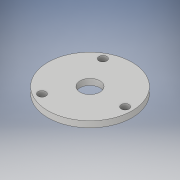
# Autodesk Inventor part: disk-sheet-b
Saved by Autodesk Inventor 2019.4 (Build 234330000, 330)
## iProperties
Created: 2020-04-05
Part Number: disk-sheet-b
Material: Generic
Document SubType Name: Sheet Metal
Designer: Phil
Density: 1 g/cm^3
Sheet Metal Rule: Default
Appearance: Default
Sheet Metal Width: 1.650 in
Sheet Metal Length: 1.650 in
Sheet Metal Area: 2.723 in^2
Flat Pattern Width: 4.191 cm
Flat Pattern Length: 4.191 cm
Flat Pattern Area: 17.5645 cm^2
Author: Phil
Autodesk Inventor part; units mm, degrees
ref_plane "YZ Plane" through (0, 0, 0) normal (1, 0, 0) x (0, 1, 0)
ref_plane "XZ Plane" through (0, 0, 0) normal (0, 1, 0) x (-1, 0, 0)
ref_plane "XY Plane" through (0, 0, 0) normal (0, 0, 1) x (1, 0, 0)
sketch "Sketch1" plane through (0, 0, 0) normal (0, 1, 0) x (-1, 0, 0)
  circle A0 centre (0, 0) radius 20.955
  circle A1 centre (0, 0) radius 4.9606
  circle A2 centre (-17.5514, 0) radius 1.9812
  circle A3 centre (8.7757, -15.2) radius 1.9812
  circle A4 centre (8.7757, 15.2) radius 1.9812
  dimension "d0" = 41.91
  dimension "d1" = 9.9212
  dimension "d2" = 3.9624
  dimension "d5" = 360
  measures "d0" diameter of A0
  measures "d1" diameter of A1
  measures "d2" diameter of A2
extrude "Plate1" add sketch "Sketch1" along normal blind 3.048
equation "\"d7\" = Thickness"
equation "\"BendRadius\" = Thickness"
equation "\"BendReliefWidth\" = Thickness"
equation "\"BendReliefDepth\" = 0.5 * Thickness"
equation "\"CornerReliefSize\" = 4 * Thickness"
equation "\"MinimumRemnant\" = 2 * Thickness"
equation "\"TransitionRadius\" = BendRadius"
equation "\"JacobiRadiusSize\" = BendRadius"
equation "\"GapSize\" = Thickness"
equation "\"Thickness\" = 3.048"
body "Solid1"
